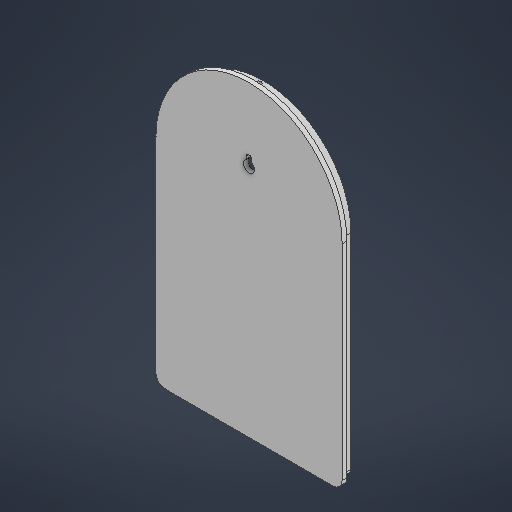
# Autodesk Inventor part: lid
Saved by Autodesk Inventor 2026.1 (Build 301233020, 233B)
## iProperties
Created: 2025-12-06
Part Number: lid
Material: Generic
Document SubType Name: Modeling
Designer: ASUS
Density: 1 g/cm^3
Appearance: Default
Author: ASUS
Autodesk Inventor part; units mm, degrees
ref_plane "YZ Plane" through (0, 0, 0) normal (1, 0, 0) x (0, 1, 0)
ref_plane "XZ Plane" through (0, 0, 0) normal (0, 1, 0) x (-1, 0, 0)
ref_plane "XY Plane" through (0, 0, 0) normal (0, 0, 1) x (1, 0, 0)
sketch "Sketch1" plane through (0, 0, 0) normal (0, 0, 1) x (1, 0, 0)
  line L0 (50, -70) -> (50, 25)
  line L1 (-50, 25) -> (-50, -70)
  line L2 (0, 0) -> (-38.1854, 57.2781) construction
  arc A0 (50, 25) -> (-50, 25) centre (0, 25) ccw
  line L3 (-45, -90) -> (45, -90)
  line L4 (0, 0) -> (38.1854, 57.2781) construction
  line L5 (50, -70) -> (50, -85)
  line L6 (-50, -70) -> (-50, -85)
  arc A1 (45, -90) -> (50, -85) centre (45, -85) ccw
  arc A2 (-50, -85) -> (-45, -90) centre (-45, -85) ccw
  line L7 (-47.25, 25) -> (-47.25, -70)
  line L8 (-47.25, -70) -> (-47.25, -85)
  arc A3 (-47.25, -85) -> (-45, -87.25) centre (-45, -85) ccw
  line L9 (-45, -87.25) -> (45, -87.25)
  arc A4 (45, -87.25) -> (47.25, -85) centre (45, -85) ccw
  line L10 (47.25, -85) -> (47.25, -70)
  line L11 (47.25, -70) -> (47.25, 25)
  arc A5 (47.25, 25) -> (-47.25, 25) centre (0, 25) ccw
  dimension "d0" = 5
  dimension "d1" = 2.75
  constraints: 24 end point, 14 point on circle, 6 centre point, 6 tangent, 2 parallel, 2 vertical, 1 equal radius, 7 other
  measures "d0" radius of A1
  measures "d1" radial gap between concentric circles of A0 A5
extrude "Extrusion1" add sketch "Sketch1" along normal blind 2.5 contours L5 A1 L3 A2 L6 L1 A0 L0 | A5 L11 L10 A4 L9 A3 L8 L7
sketch "Sketch2" plane through (0, 0, 0) normal (0, 0, -1) x (-1, 0, 0)
  line L0 (50, -70) -> (50, 25)
  line L1 (-50, 25) -> (-50, -70)
  line L2 (0, 0) -> (-38.1854, 57.2781) construction
  arc A0 (50, 25) -> (-50, 25) centre (0, 25) ccw
  line L3 (-45, -90) -> (45, -90)
  line L4 (0, 0) -> (38.1854, 57.2781) construction
  line L5 (50, -70) -> (50, -85)
  line L6 (-50, -70) -> (-50, -85)
  arc A1 (45, -90) -> (50, -85) centre (45, -85) ccw
  arc A2 (-50, -85) -> (-45, -90) centre (-45, -85) ccw
  line L7 (-47.25, 25) -> (-47.25, -70)
  line L8 (-47.25, -70) -> (-47.25, -85)
  arc A3 (-47.25, -85) -> (-45, -87.25) centre (-45, -85) ccw
  line L9 (-45, -87.25) -> (45, -87.25)
  arc A4 (45, -87.25) -> (47.25, -85) centre (45, -85) ccw
  line L10 (47.25, -85) -> (47.25, -70)
  line L11 (47.25, -70) -> (47.25, 25)
  arc A5 (47.25, 25) -> (-47.25, 25) centre (0, 25) ccw
  line L12 (-45.25, 25) -> (-45.25, -70)
  line L13 (-45.25, -70) -> (-45.25, -85)
  arc A6 (-45.25, -85) -> (-45, -85.25) centre (-45, -85) ccw
  line L14 (-45, -85.25) -> (45, -85.25)
  arc A7 (45, -85.25) -> (45.25, -85) centre (45, -85) ccw
  line L15 (45.25, -85) -> (45.25, -70)
  line L16 (45.25, -70) -> (45.25, 25)
  arc A8 (45.25, 25) -> (-45.25, 25) centre (0, 25) ccw
  line L17 (-5, -80.25) -> (5, -80.25)
  line L18 (-5, -85.25) -> (-5, -80.25)
  line L19 (5, -80.25) -> (5, -85.25)
  line L20 (-5, 65.25) -> (5, 65.25)
  line L21 (-5, 69.9729) -> (-5, 65.25)
  line L22 (5, 65.25) -> (5, 69.9729)
  dimension "d4" = 5
  dimension "d5" = 2.75
  dimension "d6" = 2
  constraints: 46 end point, 22 point on circle, 9 centre point, 6 tangent, 4 parallel, 2 point on line, 2 vertical, 1 equal radius, 14 other
  measures "d4" radius of A1
  measures "d5" radial gap between concentric circles of A0 A5
  measures "d6" radial gap between concentric circles of A5 A8
extrude "Extrusion2" add sketch "Sketch2" along normal blind 5 contours A5 L11 L10 A4 L9 A3 L8 L7 | A8 L22 L20 L21 | L18 L17 L19 L14
sketch "Sketch3" plane through (-45, -87.25, 0) normal (0, -1, 0) x (1, 0, 0)
  line L0 (45, 0) -> (45, -5)
  line L1 (-2.25, -5) -> (92.25, -5) projected
  circle A0 centre (45, -2.5) radius 1.45
  line L2 (0, 0) -> (90, 0) projected
  dimension "d10" = 2.9
  dimension "d16" = 5
  constraints: 2 end point, 2 midpoint, 1 centre point
  measures "d10" diameter of A0
  measures "d16" distance between parallel lines of L2 L1
extrude "Extrusion3" cut sketch "Sketch3" against normal through all
sketch "Sketch4" plane through (0, 0, 0) normal (0, 0, -1) x (-1, 0, 0)
  arc A0 (-1.5, 38.5981) -> (1.5, 38.5981) centre (0, 36) ccw
  arc A1 (1.5, 40) -> (-1.5, 40) centre (0, 40) ccw
  line L0 (-1.5, 40) -> (-1.5, 38.5981)
  line L1 (1.5, 40) -> (1.5, 38.5981)
  point P0 (0, 0)
  dimension "d13" = 3
  constraints: 4 end point, 4 point on circle, 2 centre point, 1 tangent, 1 vertical
  measures "d13" diameter of A1
extrude "Extrusion4" cut sketch "Sketch4" against normal blind 10
body "Solid1"
